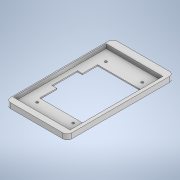
# Autodesk Inventor part: Front
Saved by Autodesk Inventor 2021 (Build 250183000, 183)
## iProperties
Created: 2021-06-27
Part Number: Front
Material: Generic
Document SubType Name: Modeling
Designer: Anton
Density: 1 g/cm^3
Appearance: Default
Author: Anton
Autodesk Inventor part; units mm, degrees
ref_plane "YZ Plane" through (0, 0, 0) normal (1, 0, 0) x (0, 1, 0)
ref_plane "XZ Plane" through (0, 0, 0) normal (0, 1, 0) x (-1, 0, 0)
ref_plane "XY Plane" through (0, 0, 0) normal (0, 0, 1) x (1, 0, 0)
sketch "Sketch1" plane through (0, 0, 0) normal (0, 1, 0) x (-1, 0, 0)
  line L0 (8, 0) -> (102.94, 0)
  line L1 (110.94, -8) -> (110.94, -185.2)
  line L2 (102.94, -193.2) -> (8, -193.2)
  line L3 (0, -185.2) -> (0, -8)
  circle A0 centre (86.7029, -32) radius 2.1
  circle A1 centre (88.297, -158.2) radius 2.1
  circle A2 centre (22.6, -158.501) radius 2.1
  circle A3 centre (21.4029, -32) radius 2.1
  arc A4 (110.94, -8) -> (102.94, 0) centre (102.94, -8) ccw
  arc A5 (8, 0) -> (0, -8) centre (8, -8) ccw
  arc A6 (0, -185.2) -> (8, -193.2) centre (8, -185.2) ccw
  arc A7 (102.94, -193.2) -> (110.94, -185.2) centre (102.94, -185.2) ccw
  point P0 (0, 0)
  dimension "d0" = 110.94
  dimension "d1" = 193.2
  dimension "d2" = 4.2
  dimension "d3" = 4.2
  dimension "d4" = 65.3
  dimension "d5" = 65.697
  dimension "d6" = 4.2
  dimension "d7" = 4.2
  dimension "d8" = 126.2
  dimension "d9" = 126.501
  dimension "d10" = 0
  dimension "d11" = 22.6
  dimension "d12" = 35
  dimension "d13" = 8
  constraints: 8 centre point, 8 end point, 8 point on circle, 8 tangent, 3 equal radius, 2 parallel, 2 point on line, 1 horizontal, 1 perpendicular
  measures "d0" distance between parallel lines of L3 L1
  measures "d1" distance between parallel lines of L2 L0
  measures "d2" diameter of A0
  measures "d3" diameter of A3
  measures "d4" distance of A3.centre A0.centre
  measures "d5" horizontal distance of A2.centre A1.centre
  measures "d6" diameter of A1
  measures "d7" diameter of A2
  measures "d8" vertical distance of A1.centre A0.centre
  measures "d9" vertical distance of A2.centre A3.centre
  measures "d10" vertical distance of A0.centre A3.centre
  measures "d11" distance from line of L3 A2.centre
  measures "d12" distance from line of L2 A1.centre
  measures "d13" radius of A4
extrude "Extrusion1" add sketch "Sketch1" along normal blind 2
sketch "Sketch2" plane through (0, 2, 0) normal (0, 1, 0) x (1, 0, 0)
  line L0 (-8, 193.2) -> (-102.94, 193.2) projected
  arc A0 (-102.94, 193.2) -> (-110.94, 185.2) centre (-102.94, 185.2) ccw projected
  line L1 (-110.94, 185.2) -> (-110.94, 8) projected
  arc A1 (-110.94, 8) -> (-102.94, 0) centre (-102.94, 8) ccw projected
  line L2 (-102.94, 0) -> (-8, 0) projected
  arc A2 (-8, 0) -> (0, 8) centre (-8, 8) ccw projected
  line L3 (0, 8) -> (0, 185.2) projected
  arc A3 (0, 185.2) -> (-8, 193.2) centre (-8, 185.2) ccw projected
  circle A4 centre (-86.7029, 32) radius 2.1 projected
  circle A5 centre (-88.297, 158.2) radius 2.1 projected
  circle A6 centre (-22.6, 158.501) radius 2.1 projected
  circle A7 centre (-21.4029, 32) radius 2.1 projected
  line L4 (-108.94, 11) -> (-108.94, 179.2)
  line L5 (-108.94, 179.2) -> (-6, 179.2)
  line L6 (-6, 11) -> (-108.94, 11)
  line L7 (-6, 179.2) -> (-6, 11)
  point P0 (0, 0)
  dimension "d16" = 2
  dimension "d17" = 14
  dimension "d18" = 11
  dimension "d19" = 6
  constraints: 8 end point, 1 horizontal
  measures "d16" distance between parallel lines of L1 L4
  measures "d17" distance between parallel lines of L0 L5
  measures "d18" distance between parallel lines of L2 L6
  measures "d19" distance between parallel lines of L3 L7
extrude "Extrusion2" add sketch "Sketch2" along normal blind 7.5 contours A3 L3 A2 L2 A1 L1 A0 L0
sketch "Sketch3" plane through (0, 2, 0) normal (0, 1, 0) x (1, 0, 0)
  line L0 (-91, 41) -> (-12, 41)
  line L1 (-12, 41) -> (-12, 146)
  line L2 (-12, 146) -> (-91, 146)
  line L3 (-6, 179.2) -> (-6, 11) projected
  line L4 (-6, 11) -> (-108.94, 11) projected
  line L5 (-99.94, 72) -> (-91, 72)
  line L6 (-91, 118.2) -> (-99.94, 118.2)
  line L7 (-99.94, 118.2) -> (-99.94, 72)
  circle A0 centre (-88.297, 158.2) radius 2.1 projected
  circle A1 centre (-86.7029, 32) radius 2.1 projected
  line L8 (-108.94, 11) -> (-108.94, 179.2) projected
  line L9 (-91, 146) -> (-91, 118.2)
  line L10 (-91, 72) -> (-91, 41)
  point P0 (0, 0)
  dimension "d22" = 105
  dimension "d24" = 6
  dimension "d25" = 30
  dimension "d26" = 40
  dimension "d27" = 40
  dimension "d28" = 9
  constraints: 16 end point, 4 parallel, 2 horizontal, 1 perpendicular
  measures "d22" distance between parallel lines of L2 L0
  measures "d24" distance between parallel lines of L3 L1
  measures "d25" distance between parallel lines of L4 L0
  measures "d26" distance from line of L6 A0.centre
  measures "d27" distance from line of L5 A1.centre
  measures "d28" distance between parallel lines of L8 L7
extrude "Extrusion3" cut sketch "Sketch3" against normal blind 7.5 contours L10 L5 L7 L6 L9 L2 L1 L0
body "Solid1"
